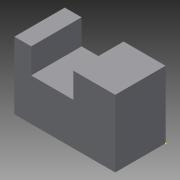
# Autodesk Inventor part: 4.1e Q2
Saved by Autodesk Inventor 2015 (Build 190159000, 159)
## iProperties
Created: 2017-11-13
Part Number: 4.1e Q2
Material: Generic
Document SubType Name: Modeling
Designer: Administrator
Density: 1 g/cm^3
Appearance: Default
Author: Administrator
Autodesk Inventor part; units mm, degrees
ref_plane "YZ Plane" through (0, 0, 0) normal (1, 0, 0) x (0, 1, 0)
ref_plane "XZ Plane" through (0, 0, 0) normal (0, 1, 0) x (-1, 0, 0)
ref_plane "XY Plane" through (0, 0, 0) normal (0, 0, 1) x (1, 0, 0)
sketch "Sketch1" plane through (0, 0, 0) normal (0, 0, 1) x (1, 0, 0)
  line L0 (0, 0) -> (0, 1016)
  line L1 (0, 1016) -> (254, 1016)
  line L2 (254, 1016) -> (254, 635)
  line L3 (254, 635) -> (889, 635)
  line L4 (889, 635) -> (889, 1016)
  line L5 (889, 1016) -> (1524, 1016)
  line L6 (1524, 1016) -> (1524, 0)
  line L7 (1524, 0) -> (0, 0)
  dimension "d0" = 1016
  dimension "d1" = 1524
  dimension "d2" = 1016
  dimension "d3" = 381
  dimension "d4" = 254
  dimension "d5" = 635
  constraints: 16 end point, 7 perpendicular, 1 vertical
  measures "d0" distance of L0.start L0.end
  measures "d1" distance of L6.end L0.start
  measures "d2" distance of L5.end L6.end
  measures "d3" distance of L1.end L2.end
  measures "d4" distance of L0.end L1.end
  measures "d5" distance of L4.end L5.end
extrude "Extrusion1" add sketch "Sketch1" along normal blind 762
sketch "Sketch2" plane through (1524, 0, 0) normal (1, 0, 0) x (0, 0, -1)
  point P0 (0, 0)
body "Solid1"
